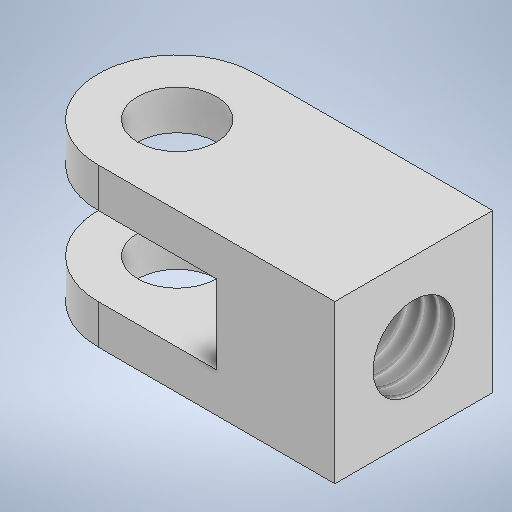
# Autodesk Inventor part: 207 part 2
Saved by Autodesk Inventor 2025.1 (Build 291241000, 241)
## iProperties
Created: 2024-08-23
Part Number: 207 part 2
Material: Generisch
Document SubType Name: Modeling
Designer: ffogue
Density: 1 g/cm^3
Appearance: Vorgabe
Author: ffogue
Autodesk Inventor part; units mm, degrees
ref_plane "YZ Plane" through (0, 0, 0) normal (1, 0, 0) x (0, 1, 0)
ref_plane "XZ Plane" through (0, 0, 0) normal (0, 1, 0) x (-1, 0, 0)
ref_plane "XY Plane" through (0, 0, 0) normal (0, 0, 1) x (1, 0, 0)
sketch "Sketch1" plane through (0, 0, 0) normal (0, 0, 1) x (1, 0, 0)
  line L0 (0, 4) -> (-12, 4)
  line L1 (-12, -4) -> (0, -4)
  line L2 (0, -4) -> (0, 4)
  arc A0 (-12, 4) -> (-12, -4) centre (-12, 0) ccw
  point P0 (0, 0)
  point P1 (0, 0)
  dimension "d0" = 4
  dimension "d1" = 12
  dimension "d2" = 8
  constraints: 6 end point, 2 point on circle, 2 tangent, 1 centre point, 1 coincident, 1 horizontal, 1 horizontal alignment, 1 midpoint, 1 parallel
  measures "d0" radius of A0
  measures "d1" distance from line of L2 A0.centre
  measures "d2" distance of L1.end L0.start
extrude "Extrusion1" add sketch "Sketch1" along normal mid plane 8
sketch "Sketch3" plane through (0, 0, 4) normal (0, 0, 1) x (1, 0, 0)
  arc A0 (-12, 4) -> (-12, -4) centre (-12, 0) ccw projected
  point P0 (0, 0)
  point P1 (-12, 0)
  constraints: 1 coincident
hole "Hole1" at (-12, 0, 4) direction (0, 0, -1) diameter 4 depth 8
sketch "Sketch2" plane through (-12, 4, 4) normal (0, 1, 0) x (1, 0, 0)
  line L0 (-4, 6) -> (6, 6)
  line L1 (6, 6) -> (6, 2)
  line L2 (6, 2) -> (-4, 2)
  line L3 (-4, 2) -> (-4, 6)
  line L4 (12, 8) -> (12, 0) projected
  line L5 (-4, 8) -> (-4, 0) projected
  point P0 (12, 4)
  point P1 (12, 4)
  point P2 (-4, 4)
  dimension "d5" = 10
  dimension "d6" = 4
  constraints: 8 end point, 3 midpoint, 2 parallel, 1 horizontal, 1 horizontal alignment, 1 perpendicular
  measures "d5" distance between parallel lines of L3 L1
  measures "d6" distance between parallel lines of L2 L0
extrude "Extrusion2" cut sketch "Sketch2" against normal up to surface (8 mm away)
sketch "Sketch4" plane through (0, -4, 4) normal (1, 0, 0) x (0, 0, -1)
  point P0 (4, 4)
  point P1 (4, 4)
  constraints: 1 coincident
hole "Hole2" at (0, 0, 0) direction (-1, 0, 0) diameter 4.134 depth 6 thread size "M5x0.8" class "6H" standard "ISO Metric profile"
body "Solid1"
